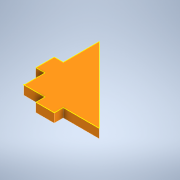
# Autodesk Inventor part: chassis_1_4
Saved by Autodesk Inventor 2022 (Build 260153000, 153)
## iProperties
Created: 2023-03-24
Part Number: chassis_1_4
Material: 一般
Document SubType Name: Modeling
Designer: Johnny Jou
Density: 1 g/cm^3
Appearance: 橙
Author: Johnny Jou
Autodesk Inventor part; units mm, degrees
ref_plane "YZ Plane" through (0, 0, 0) normal (1, 0, 0) x (0, 1, 0)
ref_plane "XZ Plane" through (0, 0, 0) normal (0, 1, 0) x (-1, 0, 0)
ref_plane "XY Plane" through (0, 0, 0) normal (0, 0, 1) x (1, 0, 0)
sketch "草圖1" plane through (0, 0, 0) normal (0, 1, 0) x (-1, 0, 0)
  line L0 (0, 0) -> (0, -25)
  line L1 (0, -25) -> (-25, 0)
  line L2 (-25, 0) -> (0, 0)
  line L3 (0, -6.95) -> (3, -6.95)
  line L4 (3, -6.95) -> (3, -13.05)
  line L5 (3, -13.05) -> (0, -13.05)
  line L6 (0, -13.05) -> (0, -6.95)
  line L7 (-6.95, 0) -> (-13.05, 0)
  line L8 (-13.05, 0) -> (-13.05, 3)
  line L9 (-13.05, 3) -> (-6.95, 3)
  line L10 (-6.95, 3) -> (-6.95, 0)
  point P0 (0, -13.05)
  dimension "d0" = 25
  dimension "d1" = 25
  dimension "d2" = 6.95
  dimension "d3" = 6.95
  dimension "d4" = 6.1
  dimension "d5" = 6.1
  dimension "d6" = 3
  dimension "d7" = 3
  constraints: 22 end point, 4 parallel, 3 perpendicular, 2 horizontal, 2 point on line, 1 vertical
  measures "d0" distance of L0.start L0.end
  measures "d1" distance of L1.end L0.start
  measures "d2" distance between parallel lines of L2 L3
  measures "d3" distance between parallel lines of L0 L10
  measures "d4" distance of L3.end L4.end
  measures "d5" distance of L8.end L9.end
  measures "d6" distance between parallel lines of L2 L9
  measures "d7" distance between parallel lines of L0 L4
extrude "擠出1" add sketch "草圖1" along normal blind 3
sketch "草圖2" plane through (0, 3, 0) normal (0, 1, 0) x (1, 0, 0)
  line L0 (-3, 6.95) -> (0, 6.95) projected
  line L1 (0, 6.95) -> (0, 0) projected
  line L2 (0, 0) -> (6.95, 0) projected
  line L3 (6.95, 0) -> (6.95, -3) projected
  line L4 (6.95, -3) -> (13.05, -3) projected
  line L5 (13.05, -3) -> (13.05, 0) projected
  line L6 (13.05, 0) -> (25, 0) projected
  line L7 (25, 0) -> (0, 25) projected
  line L8 (0, 25) -> (0, 13.05) projected
  line L9 (0, 13.05) -> (-3, 13.05) projected
  line L10 (-3, 13.05) -> (-3, 6.95) projected
equation "\"d3\" = d2"
equation "\"d5\" = d4"
